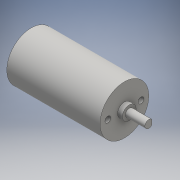
# Autodesk Inventor part: small motor
Saved by Autodesk Inventor 2016 (Build 200138000, 138)
## iProperties
Created: 2015-09-29
Part Number: small motor
Material: Generic
Document SubType Name: Modeling
Designer: Hulbert Office
Density: 1 g/cm^3
Appearance: Default
Author: Hulbert Office
Autodesk Inventor part; units mm, degrees
ref_plane "YZ Plane" through (0, 0, 0) normal (1, 0, 0) x (0, 1, 0)
ref_plane "XZ Plane" through (0, 0, 0) normal (0, 1, 0) x (-1, 0, 0)
ref_plane "XY Plane" through (0, 0, 0) normal (0, 0, 1) x (1, 0, 0)
sketch "Sketch1" plane through (0, 0, 0) normal (1, 0, 0) x (0, 1, 0)
  circle A0 centre (0, 0) radius 12.5
  dimension "d0" = 25
  constraints: 1 centre point, 1 coincident
  measures "d0" diameter of A0
extrude "Extrusion1" add sketch "Sketch1" along normal blind 47.8
sketch "Sketch2" plane through (47.8, 0, 0) normal (1, 0, 0) x (0, 0, -1)
  circle A0 centre (0, -8.5) radius 1.5
  circle A1 centre (0, 8.5) radius 1.5
  circle A2 centre (0, 0) radius 3.5
  dimension "d4" = 3
  dimension "d5" = 7
  constraints: 3 centre point, 1 coincident
  measures "d4" diameter of A0
  measures "d5" diameter of A2
extrude "Extrusion2" add sketch "Sketch2" along normal blind 2.5 contours A2
extrude "Extrusion3" cut sketch "Sketch2" against normal blind 2 contours A0 | A1
sketch "Sketch3" plane through (50.3, 0, 0) normal (1, 0, 0) x (0, 0, -1)
  circle A0 centre (0, 0) radius 2
  dimension "d10" = 4
  constraints: 1 centre point, 1 coincident
  measures "d10" diameter of A0
extrude "Extrusion4" add sketch "Sketch3" along normal blind 10
sketch "Sketch4" plane through (60.3, 0, 0) normal (1, 0, 0) x (0, 0, -1)
  circle A0 centre (0, 0) radius 2 projected
  line L0 (0, -2) -> (0, 1.5)
  line L1 (0, 1.5) -> (1.3229, 1.5)
  line L2 (-1.3229, 1.5) -> (0, 1.5)
  arc A1 (1.3229, 1.5) -> (-1.3229, 1.5) centre (0, 0) ccw
  dimension "d13" = 3.5
  constraints: 6 end point, 5 point on circle, 1 centre point, 1 collinear, 1 concentric, 1 horizontal, 1 point on line, 1 vertical
  measures "d13" distance of L0.start L0.end
extrude "Extrusion5" cut sketch "Sketch4" against normal blind 8 contours L1 L2 A0
body "Solid1"
